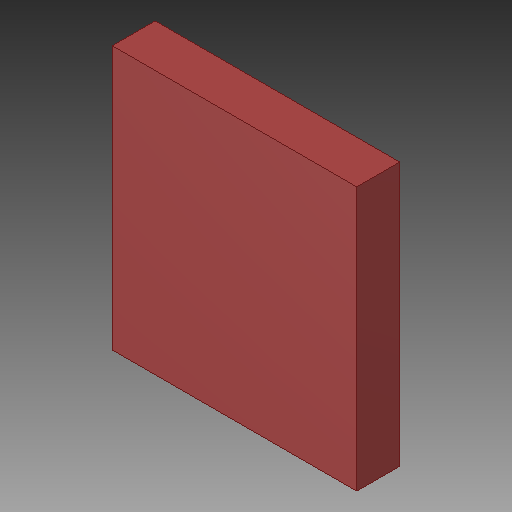
# Autodesk Inventor part: TSOP14340
Saved by Autodesk Inventor 2017 (Build 210142000, 142)
## iProperties
Created: 2019-06-13
Part Number: TSOP14340
Material: Generic
Document SubType Name: Modeling
Designer: Marc
Density: 1 g/cm^3
Appearance: TSOP143XX, TSOP14340
Author: Marc
Autodesk Inventor part; units mm, degrees
ref_plane "YZ Plane" through (0, 0, 0) normal (1, 0, 0) x (0, 1, 0)
ref_plane "XZ Plane" through (0, 0, 0) normal (0, 1, 0) x (-1, 0, 0)
ref_plane "XY Plane" through (0, 0, 0) normal (0, 0, 1) x (1, 0, 0)
sketch "TSOP143XX, TSOP14340_101" plane through (0, 0, 0) normal (0, 0, 1) x (1, 0, 0)
  line L0 (-2.6035, 3.0635) -> (3.0823, 3.0635)
  line L1 (3.0823, 3.0635) -> (3.0823, -3.0635)
  line L2 (3.0823, -3.0635) -> (-2.6035, -3.0635)
  line L3 (-2.6035, -3.0635) -> (-2.6035, 3.0635)
  constraints: 8 end point
extrude "Extrusion1" add sketch "TSOP143XX, TSOP14340_101" along normal blind 1
body "Solid1"
